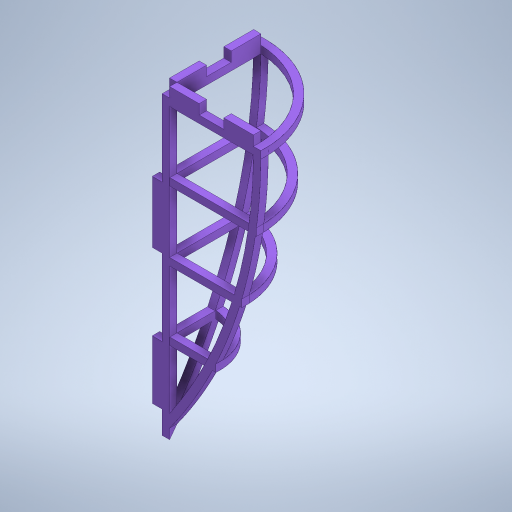
# Autodesk Inventor part: парус2
Saved by Autodesk Inventor 2023 (Build 270158000, 158)
## iProperties
Created: 2025-02-04
Part Number: парус2
Material: Типовые
Document SubType Name: Modeling
Designer: baranovaem
Density: 1 g/cm^3
Appearance: Фиолетовый
Author: baranovaem
Autodesk Inventor part; units mm, degrees
ref_plane "РабПлоскость1" through (0, 0, 0) normal (0, 0, 1) x (-1, 0, 0)
sketch "Эскиз1" plane through (0, 0, 0) normal (0, 0, 1) x (-1, 0, 0)
  line L0 (0, 0) -> (0, 120)
  line L1 (0, 0) -> (-40, 0)
  arc A0 (0, 120) -> (-40, 0) centre (154.992857, 1.669048) ccw
  line L2 (-37.00253, 3) -> (-3, 3)
  line L3 (-3, 3) -> (-3, 110.766514)
  arc A1 (-3, 110.766514) -> (-37.00253, 3) centre (154.992857, 1.669048) ccw
  dimension "d0" = 120
  dimension "d1" = 40
  dimension "d6" = 195
  dimension "d7" = 3
  constraints: 8 end point, 4 point on circle, 2 centre point, 1 horizontal, 1 vertical, 2 other
  measures "d0" distance of L0.start L0.end
  measures "d1" distance of L0.start L1.end
  measures "d6" radius of A0
  measures "d7" radial gap between concentric circles of A0 A1
sketch "Эскиз1 outline for Выдавливание1" plane through (0, 0, 0) normal (0, 0, 1) x (-1, 0, 0)
  line L0 (0, 0) -> (0, 120)
  line L1 (-40, 0) -> (0, 0)
  arc A0 (0, 120) -> (-40, 0) centre (154.992857, 1.669048) ccw
  arc A1 (-37.00253, 3) -> (-3, 110.766514) centre (154.992857, 1.669048) cw
  line L2 (-3, 3) -> (-37.00253, 3)
  line L3 (-3, 110.766514) -> (-3, 3)
extrude "Выдавливание1" add sketch "Эскиз1 outline for Выдавливание1" along normal blind 3
sketch "Эскиз2" plane through (0, 0, 0) normal (1, 0, 0) x (0, 1, 0)
  line L0 (0, 3) -> (-120, 3)
  line L1 (0, 0) -> (0, 3)
  line L2 (0, 3) -> (0, -37)
  line L3 (0, 3) -> (-120, 3)
  arc A0 (-120, 3) -> (0, -37) centre (-1.669048, 157.992857) ccw
  line L4 (-3, -34.00253) -> (-3, 0)
  line L5 (-3, 0) -> (-110.766514, 0)
  arc A1 (-110.766514, 0) -> (-3, -34.00253) centre (-1.669048, 157.992857) ccw
  dimension "d5" = 40
  dimension "d8" = 195
  dimension "d9" = 3
  constraints: 8 end point, 4 point on circle, 2 centre point, 1 vertical, 2 other
  measures "d5" distance of L0.start L2.end
  measures "d8" radius of A0
  measures "d9" radial gap between concentric circles of A0 A1
sketch "Эскиз2 outline for Выдавливание2" plane through (0, 0, 0) normal (1, 0, 0) x (0, 1, 0)
  arc A0 (-120, 3) -> (0, -37) centre (-1.669048, 157.992857) ccw
  line L0 (0, 3) -> (-120, 3)
  line L1 (0, -37) -> (0, 0)
  line L2 (0, 0) -> (0, 3)
  arc A1 (-3, -34.00253) -> (-110.766514, 0) centre (-1.669048, 157.992857) cw
  line L3 (-3, 0) -> (-3, -34.00253)
  line L4 (-110.766514, 0) -> (-3, 0)
extrude "Выдавливание2" add sketch "Эскиз2 outline for Выдавливание2" along normal blind 3
sketch "Эскиз3" plane through (0, 0, 0) normal (0, 1, 0) x (-1, 0, 0)
  line L0 (-40.007143, 0) -> (-40.007143, 3)
  arc A0 (-40.007143, 3) -> (0, -37) centre (-1.5, 1.506876) ccw
  arc A1 (-37.004698, 3) -> (0, -33.997532) centre (-1.5, 1.506876) ccw
  line L1 (0, -37) -> (0, 3)
  line L2 (0, -33.997532) -> (0, -37)
  line L3 (-37.004698, 3) -> (-40.007143, 3)
  line L4 (-3, 0) -> (-37.00253, 0)
  point P0 (0, 0)
  point P1 (0, -33.997532)
  point P2 (-3, -37)
  dimension "d13" = 3
  dimension "d18" = 38.53608
  constraints: 5 point on circle, 4 end point, 2 centre point, 1 parallel, 1 point on line, 1 vertical
  measures "d13" radial gap between concentric circles of A0 A1
  measures "d18" radius of A0
sketch "Эскиз3 outline for Выдавливание3" plane through (0, 0, 0) normal (0, 1, 0) x (-1, 0, 0)
  arc A0 (-40.007143, 3) -> (0, -37) centre (-1.5, 1.506876) ccw
  line L0 (-37.004698, 3) -> (-40.007143, 3)
  arc A1 (0, -33.997532) -> (-37.004698, 3) centre (-1.5, 1.506876) cw
  line L1 (0, -37) -> (0, -33.997532)
extrude "Выдавливание3" add sketch "Эскиз3 outline for Выдавливание3" against normal blind 3
ref_plane "РабПлоскость2" through (3, -28, 3) normal (0, -1, 0) x (1, 0, 0)
sketch "Эскиз4" plane through (3, -28, 3) normal (0, -1, 0) x (1, 0, 0)
  line L0 (35.221224, 0) -> (35.221224, -3)
  line L1 (35.221224, -3) -> (32.193055, -3)
  line L2 (32.193055, -3) -> (32.193055, 0)
  line L3 (32.193055, 0) -> (35.221224, 0)
  line L4 (0, -38.221224) -> (-3, -38.221224)
  line L5 (-3, -38.221224) -> (-3, -35.193055)
  line L6 (-3, -35.193055) -> (0, -35.193055)
  line L7 (0, -35.193055) -> (0, -38.221224)
  line L8 (-3, 0) -> (0, 0)
  line L9 (0, -0.093866) -> (0, -3)
  line L10 (0, -3) -> (-3, -3)
  line L11 (-3, -3) -> (-3, 0)
  arc A0 (-3, -38.221224) -> (35.221224, 0) centre (-1.5, -1.5) ccw
  arc A1 (-3, -35.218499) -> (32.222544, -0.093866) centre (-1.5, -1.5) ccw
  line L12 (-3, -3) -> (-3, -35.218499)
  line L13 (-3, -3) -> (-3, -37.00253)
  line L14 (0, -3) -> (0, -35.193055)
  line L15 (0, -3) -> (32.193055, -3)
  line L16 (34.00253, -3) -> (34.00253, 0)
  line L17 (32.222544, -0.093866) -> (0, -0.093866)
  line L18 (-3, 0) -> (37.007143, 0)
  point P0 (32.218499, -3)
  point P1 (0, -35.218499)
  point P2 (35.221224, -3)
  point P3 (32.193055, -0.093866)
  dimension "d24" = 3
  constraints: 8 end point, 5 point on circle, 2 centre point, 1 collinear, 1 horizontal, 1 parallel, 1 perpendicular, 1 other
  measures "d24" radial gap between concentric circles of A0 A1
sketch "Эскиз4 outline for Выдавливание5" plane through (3, -28, 3) normal (0, -1, 0) x (1, 0, 0)
  arc A0 (32.218499, -3) -> (0, -35.218499) centre (-1.5, -1.5) cw
  line L0 (0, -35.218499) -> (0, -3)
  line L1 (0, -3) -> (32.218499, -3)
  line L2 (32.193055, 0) -> (32.193055, -0.093866)
  line L3 (32.193055, -0.093866) -> (0, -0.093866)
  line L4 (0, -0.093866) -> (-3, 0)
  line L5 (-3, 0) -> (-3, -3)
  line L6 (-3, -3) -> (-3, -38.221224)
  line L7 (-3, -38.221224) -> (0, -38.221224)
  arc A1 (0, -38.221224) -> (35.221224, -3) centre (-1.5, -1.5) ccw
  line L8 (35.221224, -3) -> (35.221224, 0)
  line L9 (35.221224, 0) -> (32.193055, 0)
extrude "Выдавливание5" add sketch "Эскиз4 outline for Выдавливание5" along normal blind 3
ref_plane "РабПлоскость3" through (3, -56, 3) normal (0, -1, 0) x (1, 0, 0)
sketch "Эскиз6" plane through (3, -56, 3) normal (0, -1, 0) x (1, 0, 0)
  line L0 (29.285406, -3) -> (26.159655, -3)
  line L1 (26.159655, -3) -> (26.159655, 0)
  line L2 (26.159655, 0) -> (29.285406, 0)
  line L3 (29.285406, 0) -> (29.285406, -3)
  line L4 (0, -29.159655) -> (0, -32.285406)
  line L5 (0, -32.285406) -> (-3, -32.285406)
  line L6 (-3, -32.285406) -> (-3, -29.159655)
  line L7 (-3, -29.159655) -> (0, -29.159655)
  line L8 (-3, 0) -> (0, 0)
  line L9 (0, 0) -> (0, -3)
  line L10 (0, -3) -> (-3, -3)
  line L11 (-3, -3) -> (-3, 0)
  arc A0 (-3, -32.285406) -> (29.285406, 0) centre (-1.5, -1.5) ccw
  arc A1 (-3, -29.281462) -> (26.281462, 0) centre (-1.5, -1.5) ccw
  line L12 (-3, -32.285406) -> (-3, -29.281462)
  line L13 (29.285406, 0) -> (26.281462, 0)
  line L14 (0, -3) -> (-3, -3)
  line L15 (-3, -3) -> (-3, -29.281462)
  line L16 (0, -3) -> (0, -36.997532)
  line L17 (0, -29.159655) -> (0, -3)
  line L18 (0, -3) -> (26.281462, -3)
  line L19 (0, -3) -> (0, 0)
  line L20 (26.281462, 0) -> (0, 0)
  point P0 (26.281462, -3)
  point P1 (0, -29.281462)
  dimension "d29" = 3
  constraints: 12 end point, 6 point on circle, 2 centre point, 2 collinear, 2 point on line, 1 horizontal, 1 perpendicular
  measures "d29" radial gap between concentric circles of A0 A1
sketch "Эскиз6 outline for Выдавливание6" plane through (3, -56, 3) normal (0, -1, 0) x (1, 0, 0)
  line L0 (0, -29.281462) -> (0, -3)
  line L1 (0, -3) -> (26.281462, -3)
  arc A0 (26.281462, -3) -> (0, -29.281462) centre (-1.5, -1.5) cw
  line L2 (29.285406, 0) -> (-3, 0)
  line L3 (-3, 0) -> (-3, -3)
  line L4 (-3, -3) -> (-3, -32.285406)
  line L5 (-3, -32.285406) -> (0, -32.285406)
  arc A1 (0, -32.285406) -> (29.285406, -3) centre (-1.5, -1.5) ccw
  line L6 (29.285406, -3) -> (29.285406, 0)
extrude "Выдавливание6" add sketch "Эскиз6 outline for Выдавливание6" along normal blind 3
ref_plane "РабПлоскость4" through (3, -84, 3) normal (0, -1, 0) x (1, 0, 0)
sketch "Эскиз7" plane through (3, -84, 3) normal (0, -1, 0) x (1, 0, 0)
  line L0 (18.774262, -3) -> (15.459195, -3)
  line L1 (15.459195, -3) -> (15.459195, 0)
  line L2 (15.459195, 0) -> (18.774262, 0)
  line L3 (18.774262, 0) -> (18.774262, -3)
  line L4 (-3, -18.459195) -> (0, -18.459195)
  line L5 (0, -18.459195) -> (0, -21.774262)
  line L6 (0, -21.774262) -> (-3, -21.774262)
  line L7 (-3, -21.774262) -> (-3, -18.459195)
  line L8 (-3, 0) -> (0, 0)
  line L9 (0, 0) -> (0, -3)
  line L10 (0, -3) -> (-3, -3)
  line L11 (-3, -3) -> (-3, 0)
  arc A0 (-3, -21.774262) -> (18.774262, 0) centre (-1.5, -1.5) ccw
  arc A1 (-3, -18.764636) -> (15.764636, 0) centre (-1.5, -1.5) ccw
  line L12 (-3, -18.764636) -> (-3, -21.774262)
  line L13 (-3, -3) -> (-3, -37.00253)
  line L14 (15.764636, 0) -> (18.774262, 0)
  line L15 (0, -3) -> (0, -36.997532)
  line L16 (0, -3) -> (0, -18.764636)
  line L17 (0, 0) -> (15.764636, 0)
  line L18 (31.75354, -0.093866) -> (0, -0.093866)
  line L19 (15.459195, -3) -> (0, -3)
  point P0 (15.459195, -0.093866)
  dimension "d33" = 3
  constraints: 10 end point, 6 point on circle, 2 centre point, 2 collinear, 2 parallel, 2 point on line
  measures "d33" radial gap between concentric circles of A0 A1
sketch "Эскиз7 outline for Выдавливание7" plane through (3, -84, 3) normal (0, -1, 0) x (1, 0, 0)
  arc A0 (15.764636, 0) -> (-3, -18.764636) centre (-1.5, -1.5) cw
  line L0 (18.774262, 0) -> (15.764636, 0)
  arc A1 (-3, -21.774262) -> (18.774262, 0) centre (-1.5, -1.5) ccw
  line L1 (-3, -18.764636) -> (-3, -21.774262)
  line L2 (0, 0) -> (-3, 0)
  line L3 (0, -0.093866) -> (0, 0)
  line L4 (15.459195, -0.093866) -> (0, -0.093866)
  line L5 (15.459195, -3) -> (15.459195, -0.093866)
  line L6 (0, -3) -> (15.459195, -3)
  line L7 (0, -18.459195) -> (0, -3)
  line L8 (-3, -18.459195) -> (0, -18.459195)
  line L9 (-3, -3) -> (-3, -18.459195)
  line L10 (-3, 0) -> (-3, -3)
extrude "Выдавливание7" add sketch "Эскиз7 outline for Выдавливание7" along normal blind 3
sketch "Эскиз8" plane through (0, 0, 3) normal (0, 1, 0) x (1, 0, 0)
  line L0 (3, 3) -> (37.004117, 3) construction
  arc A0 (37.004117, 3) -> (3, 36.997532) centre (1.5, 1.493124) ccw construction
  line L1 (3, 36.997532) -> (3, 3) construction
  line L2 (40.007143, 0) -> (0, 0) construction
  line L3 (0, 0) -> (0, 40) construction
  arc A1 (3, 40) -> (0, 40) centre (1.5, 1.493124) ccw construction
  arc A2 (40.007143, 0) -> (3, 40) centre (1.5, 1.493124) ccw construction
  line L4 (37.00253, 3) -> (37.00253, 0)
  line L5 (37.004117, 3) -> (37.00253, 0)
  line L6 (3, 3) -> (29.159655, 3)
  line L7 (15, 3) -> (15, 0)
  line L8 (29.159655, 0) -> (3, 0)
  line L9 (25, 3) -> (25, 0)
  line L10 (3, 0) -> (3, 3)
  line L11 (3, 0) -> (3, 3)
  line L12 (3, 3) -> (15, 3)
  line L13 (3, 0) -> (15, 0)
  line L14 (3, 0) -> (37.00253, 0)
  line L15 (25, 0) -> (37.00253, 0)
  line L16 (37.00253, 3) -> (35.193055, 3)
  line L17 (25, 3) -> (37.00253, 3)
  line L18 (3, 3) -> (0, 3)
  arc A3 (37.004117, 3) -> (3, 36.997532) centre (1.5, 1.493124) ccw
  line L19 (3, 36.997532) -> (0, 37.124277)
  line L20 (3, 15) -> (0, 15)
  line L21 (0, 40) -> (0, 0)
  line L22 (3, 25) -> (0, 25)
  line L23 (3, 3) -> (3, 36.997532)
  line L24 (3, 3) -> (3, 15)
  line L25 (0, 3) -> (3, 3)
  line L26 (0, 3) -> (0, 15)
  line L27 (0, 37.00253) -> (0, 35.193055)
  line L28 (0, 25) -> (0, 37.00253)
  line L29 (3, 37.00253) -> (3, 35.193055)
  line L30 (3, 25) -> (3, 37.00253)
  point P0 (15, 1.5)
  point P1 (0, 36.997532)
  point P2 (1.5, 15)
  point P3 (1.5, 25)
  dimension "d36" = 15
  dimension "d37" = 10
  dimension "d40" = 15
  dimension "d41" = 10
  constraints: 32 end point, 10 point on line, 5 collinear, 3 horizontal, 3 midpoint, 3 perpendicular, 2 vertical, 1 parallel, 1 tangent
  measures "d36" distance between parallel lines of L3 L7
  measures "d37" distance from line of L9 point (15, 1.5)
  measures "d40" distance from line of L2 point (1.5, 15)
  measures "d41" distance of point (1.5, 15) point (1.5, 25)
sketch "Эскиз8 outline for Выдавливание8" plane through (0, 0, 3) normal (0, 1, 0) x (1, 0, 0)
  line L0 (37.00253, 0) -> (37.00253, 3)
  line L1 (37.00253, 3) -> (25, 3)
  line L2 (25, 3) -> (25, 0)
  line L3 (25, 0) -> (37.00253, 0)
  line L4 (3, 3) -> (3, 0)
  line L5 (15, 3) -> (3, 3)
  line L6 (15, 0) -> (15, 3)
  line L7 (3, 0) -> (15, 0)
  line L8 (3, 25) -> (3, 36.997532)
  line L9 (0, 25) -> (3, 25)
  line L10 (0, 37.124277) -> (0, 25)
  line L11 (3, 36.997532) -> (0, 37.124277)
  line L12 (3, 3) -> (3, 15)
  line L13 (0, 3) -> (3, 3)
  line L14 (0, 15) -> (0, 3)
  line L15 (3, 15) -> (0, 15)
extrude "Выдавливание8" add sketch "Эскиз8 outline for Выдавливание8" along normal blind 4
sketch "Эскиз10" plane through (0, -120, 0) normal (-1, 0, 0) x (0, 0, 1)
  line L0 (-15.459195, 36) -> (0, 36)
  line L1 (0, 36) -> (0, 61)
  line L2 (0, 61) -> (-25.247864, 61)
  arc A0 (-25.247864, 61) -> (-15.459195, 36) centre (157.992857, 118.330952) ccw
  line L3 (0, 33) -> (-14.003156, 33)
  arc A1 (-14.003156, 33) -> (0, 9.233486) centre (157.992857, 118.330952) ccw
  line L4 (0, 9.233486) -> (0, 33)
  line L5 (-26.159655, 64) -> (0, 64)
  line L6 (0, 64) -> (0, 89)
  line L7 (0, 89) -> (-31.75354, 89)
  arc A2 (-31.75354, 89) -> (-26.159655, 64) centre (157.992857, 118.330952) ccw
  line L8 (-29.285406, 61) -> (-29.285406, 64)
  arc A3 (-34.788613, 89) -> (-29.285406, 64) centre (157.992857, 118.330952) ccw
  line L9 (-34.788613, 89) -> (-35.221224, 89)
  line L10 (-35.221224, 89) -> (-35.221224, 92)
  arc A4 (-37, 120) -> (-35.221224, 92) centre (157.992857, 118.330952) ccw
  line L11 (-37, 120) -> (-34.124277, 120)
  line L12 (-34.124277, 120) -> (-34.124277, 124)
  line L13 (-34.124277, 124) -> (-22, 124)
  line L14 (-22, 124) -> (-22, 120)
  line L15 (-22, 120) -> (-12, 120)
  line L16 (-12, 120) -> (-12, 124)
  line L17 (-12, 124) -> (0, 124)
  line L18 (0, 124) -> (0, 120)
  line L19 (0, 120) -> (3, 120)
  line L20 (3, 120) -> (3, 0)
  line L21 (3, 0) -> (0, 0)
  line L22 (0, 0) -> (0, 4.036346)
  arc A5 (-17.345754, 33) -> (0, 4.036346) centre (157.992857, 118.330952) ccw
  line L23 (-17.345754, 33) -> (-18.774262, 33)
  line L24 (-18.774262, 33) -> (-18.774262, 36)
  arc A6 (-28.388907, 61) -> (-18.774262, 36) centre (157.992857, 118.330952) ccw
  line L25 (-28.388907, 61) -> (-29.285406, 61)
  line L26 (-32.193055, 92) -> (0, 92)
  line L27 (0, 92) -> (0, 117)
  line L28 (0, 117) -> (-34.00253, 117)
  arc A7 (-34.00253, 117) -> (-32.193055, 92) centre (157.992857, 118.330952) ccw
  line L29 (0, 33) -> (0, 9.233486)
  line L30 (0, 9.233486) -> (3, 9.233486)
  line L31 (0, 33) -> (3, 33)
  line L32 (0, 36) -> (0, 61)
  line L33 (0, 36) -> (3, 36)
  line L34 (0, 61) -> (0, 64)
  line L35 (0, 61) -> (3, 61)
  line L36 (0, 64) -> (3, 64)
  line L37 (0, 64) -> (3, 64)
  line L38 (3, 64) -> (3, 89)
  line L39 (0, 89) -> (3, 89)
  line L40 (0, 89) -> (3, 89)
  line L41 (0, 92) -> (0, 117)
  line L42 (0, 92) -> (3, 92)
  line L43 (0, 117) -> (3, 117)
  line L44 (0, 117) -> (3, 117)
  line L45 (3, 117) -> (3, 92)
  line L46 (3, 92) -> (0, 92)
  line L47 (0, 92) -> (0, 117)
  line L48 (0, 64) -> (0, 89)
  line L49 (0, 36) -> (0, 61)
  line L50 (3, 61) -> (3, 36)
  line L51 (3, 61) -> (3, 9.233486)
  line L52 (0, 9.233486) -> (0, 33)
  constraints: 30 end point, 6 horizontal, 4 collinear, 1 parallel, 1 vertical, 7 other
sketch "Эскиз10 outline for Выдавливание10" plane through (0, -120, 0) normal (-1, 0, 0) x (0, 0, 1)
  line L0 (3, 33) -> (0, 33)
  line L1 (3, 9.233486) -> (3, 33)
  line L2 (0, 9.233486) -> (3, 9.233486)
  line L3 (0, 33) -> (0, 9.233486)
  line L4 (3, 89) -> (0, 89)
  line L5 (3, 64) -> (3, 89)
  line L6 (0, 64) -> (3, 64)
  line L7 (0, 89) -> (0, 64)
extrude "Выдавливание10" add sketch "Эскиз10 outline for Выдавливание10" along normal blind 4
